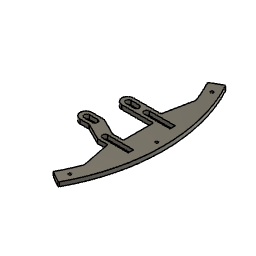
move_base_front_bumper_a (Autodesk Fusion 360 design; units mm, degrees)
Autodesk Fusion 360 part; units mm, degrees
note: some values were not read from the file. Set by a fixed rule: the direction of a hole.
sketch "スケッチ1" plane through (0, 0, 0) normal (0, 1, 0) x (1, 0, 0)
  arc A0 (181.8653, -105) -> (181.8653, 105) centre (0, 0) ccw
  line L0 (181.8653, 105) -> (0, 0)
  line L1 (0, 0) -> (181.8653, -105)
  line L2 (0, 0) -> (210, 0)
  arc A1 (168.0089, -97) -> (168.0089, 97) centre (0, 0) ccw
  line L3 (191.3426, 32) -> (135, 32)
  line L4 (135, 32) -> (135, 18)
  line L5 (135, 18) -> (193.1631, 18)
  arc A2 (165, 28.1) -> (165, 21.9) centre (165, 25) ccw
  line L6 (165, 28.1) -> (196, 28.1)
  line L7 (196, 28.1) -> (196, 21.9)
  line L8 (196, 21.9) -> (165, 21.9)
  arc A3 (143, 28.1) -> (143, 21.9) centre (143, 25) ccw
  arc A4 (153, 21.9) -> (153, 28.1) centre (153, 25) ccw
  line L9 (143, 28.1) -> (153, 28.1)
  line L10 (153, 21.9) -> (143, 21.9)
  line L11 (10, 0) -> (184.3138, 100.6401)
  arc A5 (154.1525, -89) -> (154.1525, 89) centre (0, 0) ccw
  line L12 (10, 0) -> (184.3138, -100.6401)
  line L13 (193.1631, -18) -> (167, -18)
  line L14 (163, -32) -> (191.3426, -32)
  arc A6 (133, -11.9) -> (133, -18.1) centre (133, -15) ccw
  arc A7 (143, -18.1) -> (143, -11.9) centre (143, -15) ccw
  arc A8 (165, -21.9) -> (165, -28.1) centre (165, -25) ccw
  line L15 (165, -21.9) -> (196, -21.9)
  line L16 (196, -21.9) -> (196, -28.1)
  line L17 (196, -28.1) -> (165, -28.1)
  line L18 (133, -11.9) -> (143, -11.9)
  line L19 (143, -18.1) -> (133, -18.1)
  arc A9 (183.0742, -85.3689) -> (183.0742, 85.3689) centre (0, 0) ccw
  line L20 (0, 0) -> (183.0742, 85.3689)
  line L21 (0, 0) -> (183.0742, -85.3689)
  line L22 (180, 18) -> (180, -18)
  line L23 (175.1, 32) -> (182.0632, 67)
  line L24 (175.1, -32) -> (182.0632, -67)
  line L25 (167, -18) -> (147, -8)
  line L26 (147, -8) -> (125, -8)
  line L27 (125, -8) -> (125, -22)
  line L28 (125, -22) -> (143, -22)
  line L29 (143, -22) -> (163, -32)
  point P0 (135, 25)
  point P1 (202, 0)
  point P2 (125, -15)
  dimension "d1" = 210
  dimension "d2" = 30
  dimension "d3" = 30
  dimension "d4" = 194
  dimension "d5" = 14
  dimension "d6" = 3.1
  dimension "d7" = 3.1
  dimension "d8" = 10
  dimension "d9" = 8
  dimension "d10" = 31
  dimension "d11" = 12
  dimension "d12" = 25
  dimension "d13" = 135
  dimension "d14" = 30
  dimension "d15" = 10
  dimension "d16" = 178
  dimension "d17" = 30
  dimension "d19" = 3.1
  dimension "d20" = 3.1
  dimension "d23" = 202
  dimension "d24" = 25
  dimension "d25" = 25
  dimension "d29" = 180
  dimension "d34" = 25
  dimension "d35" = 15
  dimension "d36" = 7
  dimension "d37" = 7
  dimension "d38" = 22
  dimension "d39" = 10
  dimension "d40" = 8
  dimension "d41" = 22
  dimension "d42" = 20
  dimension "d43" = 18
  dimension "d44" = 20
  dimension "d45" = 14
  dimension "d46" = 35
  dimension "d47" = 35
  constraint coincident A0.centre L0.end
  constraint coincident A0 L2.end
  constraint horizontal L2
  constraint coincident L0 A1.end
  constraint coincident L1 A1.start
  constraint coincident A1 L3.start
  constraint horizontal L3
  constraint perpendicular L3 L4
  constraint coincident A1 L5.end
  constraint perpendicular L4 L5
  constraint horizontal L6
  constraint perpendicular L6 L7
  constraint perpendicular L7 L8
  constraint tangent A2 L6
  constraint tangent A2 L8
  constraint midpoint L4 P0
  constraint horizontal A3.centre P0
  constraint horizontal A4.centre P0
  constraint horizontal A2.centre P0
  constraint tangent A3 L9
  constraint tangent A4 L9
  constraint tangent A4 L10
  constraint tangent A3 L10
  constraint horizontal L9
  constraint coincident L2 L11.start
  constraint coincident L0 A5.end
  constraint coincident A0 L11.end
  constraint coincident A0 L12.end
  constraint coincident A1 L13.start
  constraint horizontal L13
  constraint coincident A1 L14.end
  constraint parallel L13 L15
  constraint perpendicular L15 L16
  constraint perpendicular L16 L17
  constraint horizontal L18
  constraint horizontal L19
  constraint tangent A7 L18
  constraint tangent A7 L19
  constraint tangent A6 L19
  constraint tangent A6 L18
  constraint tangent A8 L15
  constraint tangent A8 L17
  constraint vertical A2.centre A8.centre
  constraint collinear L7 L16
  constraint midpoint A9 P1
  constraint coincident L5 L22.start
  constraint perpendicular L5 L22
  constraint coincident L13 L22.end
  constraint coincident L1 A5.start
  constraint coincident A5 L23.start
  constraint coincident L3 L23.start
  constraint coincident A1 L23.end
  constraint coincident A5 L24.start
  constraint coincident L14 L24.start
  constraint coincident A1 L24.end
  constraint parallel L13 L26
  constraint perpendicular L26 L27
  constraint perpendicular L27 L28
  constraint horizontal L14
  constraint midpoint L27 P2
  constraint horizontal A6.centre P2
  measures "d1" radius of A0
  measures "d2" angle of L0 L2
  measures "d3" angle of L1 L2
  measures "d4" radius of A1
  measures "d5" distance of L3.end L4.end
  measures "d6" radius of A3
  measures "d7" radius of A2
  measures "d8" distance of A3.centre A4.centre
  measures "d9" distance of L4 A3.centre
  measures "d10" distance of A2.end L7.end
  measures "d11" distance of A2.centre A4.centre
  measures "d12" vertical distance of A0.centre P0
  measures "d13" distance of A0.centre L4
  measures "d14" angle of L2 L11
  measures "d15" distance of A0.centre L11.start
  measures "d16" radius of A5
  measures "d17" angle of L2 L12
  measures "d19" radius of A6
  measures "d20" radius of A8
  measures "d23" radius of A9
  measures "d24" angle of L2 L20
  measures "d25" angle of L2 L21
  measures "d29" distance of A0.centre L22
  measures "d34" vertical distance of A0.centre A8.centre
  measures "d35" vertical distance of A0.centre A6.centre
  measures "d36" distance of L14 A8.centre
  measures "d37" distance of L13 A8.centre
  measures "d38" horizontal distance of A7.centre A8.centre
  measures "d39" distance of A6.centre A7.centre
  measures "d40" distance of A6.centre L27
  measures "d41" distance of L25.end L26.end
  measures "d42" horizontal distance of L13.end L25.end
  measures "d43" distance of L27.end L28.end
  measures "d44" horizontal distance of L14.start L28.end
  measures "d45" distance of L26.end L27.end
  measures "d46" vertical distance of L23.start L23.end
  measures "d47" vertical distance of L24.start L24.end
extrude "押し出し1" add sketch "スケッチ1" along normal blind 5 contours A0 L2 A1 L12 A9 L21 | A0 L2 A1 L11 A9 L20 | L2 A1 L15 L16 L17 A9 L21 | L2 A1 L6 L7 L8 A9 L20 | L2 A1 L13 L22 | L2 A1 L5 L22 | A1 L14 L24 | A1 A5 L13 L15 | A1 L5 L8 A5 | A1 A5 L14 L17 | A5 L13 L14 A8 L15 L17 L25 L26 L27 L28 L29 | A1 L3 L23 | L3 L4 L5 A2 L6 L8 A5 | A1 L3 L6 A5
hole "穴1" at (183.0742, 0, 85.3689) at (202, 0, 0) at (183.0742, 0, -85.3689) direction (0, 1, 0) diameter 3.2 end through all
fillet "フィレット1" radius 1 10 edges at (184.3138, 2.5, 100.6401) (184.3138, 2.5, -100.6401) (180, 2.5, -18) (180, 2.5, 18) (175.1, 2.5, 32) (175.1, 2.5, -32) (182.0632, 2.5, -67) (182.0632, 2.5, 67) (143, 2.5, 22) (167, 2.5, 18)
fillet "フィレット2" radius 7 4 edges at (135, 2.5, -18) (135, 2.5, -32) (125, 2.5, 8) (125, 2.5, 22)
